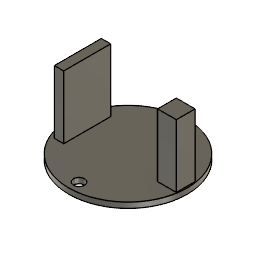
mouse-body-v115 (Autodesk Fusion 360 archive; units mm, degrees)
design "PMW3610 Breakout Board"
Autodesk Fusion 360 part; units mm, degrees
cylinder "CylinderPrimitive1" add diameter 32 height 1.5 placed x (1, 0, 0) y (0, 1, 0) z (0, 0, 1) at (0, 0, 0)
sketch "Top" plane through (0, 0, 1.5) normal (0, 0, 1) x (-1, 0, 0)
  circle A0 centre (0, 0) radius 16
  line L0 (16, 0) -> (-16, 0)
  line L1 (0, 0) -> (0, -13.225)
  line L2 (0, 0) -> (0, 13.225)
  circle A1 centre (0, -13.225) radius 1.5
  circle A2 centre (0, 13.225) radius 1.5
  line L3 (11, -20) -> (11, 20)
  line L4 (-10.5, -20) -> (-10.5, 20)
  line L5 (11, 0) -> (13.54, 0)
  line L6 (13.54, 0) -> (13.54, -6.35)
  line L7 (13.54, -6.35) -> (11, -6.35)
  line L8 (11, -6.35) -> (11, 0)
  line L9 (11, 0) -> (13.54, 0)
  line L10 (13.54, 0) -> (13.54, 6.35)
  line L11 (13.54, 6.35) -> (11, 6.35)
  line L12 (11, 6.35) -> (11, 0)
  line L13 (-10.5, 0) -> (-15.58, 0)
  line L14 (-15.58, 0) -> (-15.58, -2.54)
  line L15 (-15.58, -2.54) -> (-10.5, -2.54)
  line L16 (-10.5, -2.54) -> (-10.5, 0)
  line L17 (-10.5, 0) -> (-15.58, 0)
  line L18 (-15.58, 0) -> (-15.58, 2.54)
  line L19 (-15.58, 2.54) -> (-10.5, 2.54)
  line L20 (-10.5, 2.54) -> (-10.5, 0)
  point P0 (-16, 0)
  dimension "d6" = 13.225
  dimension "d7" = 13.225
  dimension "d8" = 3
  dimension "d9" = 3
  dimension "d12" = 11
  dimension "d13" = 10.5
  dimension "d14" = 2.54
  dimension "d15" = 6.35
  dimension "d16" = 2.54
  dimension "d17" = 6.35
  dimension "d18" = 5.08
  dimension "d19" = 2.54
  dimension "d20" = 5.08
  dimension "d21" = 2.54
  constraint coincident A0 L0.start
  constraint coincident P0 L0.end
  constraint horizontal L0
  constraint coincident A0.centre L1.start
  constraint perpendicular L0 L1
  constraint perpendicular L0 L2
  constraint coincident L1.end A1.centre
  constraint coincident L2.end A2.centre
  constraint vertical L3
  constraint vertical L4
  constraint horizontal L5
  constraint vertical L6
  constraint horizontal L7
  constraint vertical L8
  constraint midpoint L3 L5.start
  constraint horizontal L9
  constraint vertical L10
  constraint horizontal L11
  constraint vertical L12
  constraint horizontal L13
  constraint vertical L14
  constraint horizontal L15
  constraint vertical L16
  constraint midpoint L4 L13.start
  constraint horizontal L17
  constraint vertical L18
  constraint horizontal L19
  constraint vertical L20
  measures "d6" distance of A0.centre L1.end
  measures "d7" distance of A0.centre L2.end
  measures "d8" diameter of A1
  measures "d9" diameter of A2
  measures "d12" distance of L1 L3
  measures "d13" distance of L1 L4
  measures "d14" distance of L5.start L5.end
  measures "d15" distance of L5.start L7.end
  measures "d16" distance of L5.start L5.end
  measures "d17" distance of L5.start L11.end
  measures "d18" distance of L13.start L13.end
  measures "d19" distance of L13.start L15.end
  measures "d20" distance of L13.start L13.end
  measures "d21" distance of L13.start L19.end
extrude "Extrude1" cut sketch "Top" against normal blind 10 contours A1 | A2
extrude "Extrude2" add sketch "Top" along normal blind 17 contours L0 L3 L5 L6 L7 L8 L9 | L0 L3 L5 L9 L10 L11 L12 | L0 L4 L13 L17 L18 L19 L20 | L0 L4 L13 L14 L15 L16 L17
sketch "Bottom" plane through (0, 0, 0) normal (0, 0, -1) x (1, 0, 0)
  circle A0 centre (0, -13.225) radius 1.5
  circle A1 centre (0, 13.225) radius 1.5
  circle A2 centre (0, 0) radius 16
  line L0 (0, -13.225) -> (-0.0125, -11.7251)
  line L1 (-0.0125, -11.7251) -> (-0.0374, -8.7252)
  line L2 (-16, 0) -> (16, 0)
  line L3 (-0.0374, -8.7252) -> (-0.0374, -2.3902)
  line L4 (-4.0374, 3.9448) -> (3.9626, 3.9448)
  line L5 (3.9626, 3.9448) -> (3.9626, -8.7252)
  line L6 (3.9626, -8.7252) -> (-4.0374, -8.7252)
  line L7 (-4.0374, -8.7252) -> (-4.0374, 3.9448)
  line L8 (-4.0374, 3.9448) -> (3.9626, -8.7252) construction
  line L9 (3.9626, 3.9448) -> (-4.0374, -8.7252) construction
  point P0 (-0.0374, -2.3902)
  dimension "d28" = 3
  dimension "d29" = 6.335
  dimension "d30" = 8
  dimension "d31" = 12.67
  constraint coincident A0.centre L0.start
  constraint coincident A0 L0.end
  constraint parallel L0 L1
  constraint perpendicular L2 L3
  constraint horizontal L4
  constraint perpendicular L4 L5
  constraint parallel L4 L6
  constraint parallel L5 L7
  constraint coincident L8 P0
  constraint coincident L9 P0
  constraint coincident P0 L3.end
  measures "d28" distance of L0.end L1.end
  measures "d29" distance of L1.end P0
  measures "d30" distance of L5.end L6.end
  measures "d31" distance of L4.end L5.end
extrude "Extrude3" add sketch "Bottom" along normal blind 3.5 contours L2 L5 L6 L7 | L2 L4 L5 L7
equation "HOLE_SIZE = 3 mm"
equation "HOLE_SPACING = 26.45 mm"
equation "d6 = HOLE_SPACING / 2"
equation "d7 = HOLE_SPACING / 2"
equation "d8 = HOLE_SIZE"
equation "d9 = HOLE_SIZE"
equation "PLUGGED_CONNECTOR_HEIGHT = 17 mm"
equation "d23 = PLUGGED_CONNECTOR_HEIGHT"
equation "LENS_LENGTH = 12.67 mm"
equation "LENS_WIDTH = 8 mm"
equation "LENS_HEIGHT = 3.5 mm"
equation "d29 = LENS_LENGTH / 2"
equation "d30 = LENS_WIDTH"
equation "d31 = LENS_LENGTH"
equation "d32 = LENS_HEIGHT"
